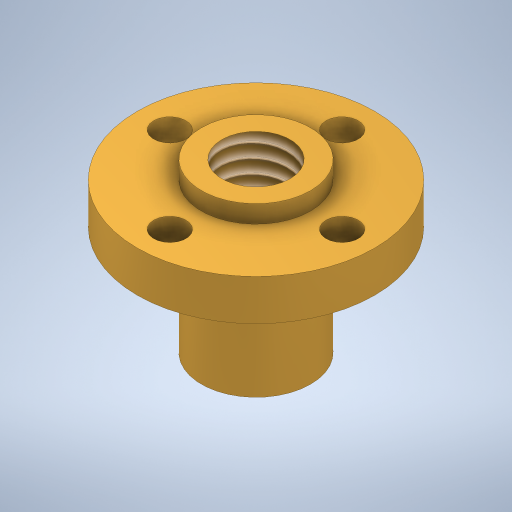
# Autodesk Inventor part: Threaded Rod Mount
Saved by Autodesk Inventor 2024 (Build 280153000, 153)
## iProperties
Created: 2023-06-07
Part Number: Threaded Rod Mount
Material: Generic
Document SubType Name: Modeling
Designer: 18179
Density: 1 g/cm^3
Appearance: Brass - Satin
Author: 18179
Autodesk Inventor part; units mm, degrees
ref_plane "YZ Plane" through (0, 0, 0) normal (1, 0, 0) x (0, 1, 0)
ref_plane "XZ Plane" through (0, 0, 0) normal (0, 1, 0) x (-1, 0, 0)
ref_plane "XY Plane" through (0, 0, 0) normal (0, 0, 1) x (1, 0, 0)
sketch "Sketch1" plane through (0, 0, 0) normal (0, 1, 0) x (-1, 0, 0)
  circle A0 centre (0, 0) radius 11.049
  circle A1 centre (0, 0) radius 3.175
  circle A2 centre (8.025, 0) radius 1.5
  line L0 (9.525, 0) -> (11.049, 0)
  circle A3 centre (0, 0) radius 5.08
  circle A4 centre (0, 8.025) radius 1.5
  circle A5 centre (-8.025, 0) radius 1.5
  circle A6 centre (0, -8.025) radius 1.5
  point P0 (0, 9.525)
  point P1 (-9.525, 0)
  point P2 (0, -9.525)
  dimension "d0" = 22.098
  dimension "d2" = 3
  dimension "d1" = 6.35
  dimension "d3" = 1.524
  dimension "d4" = 10.16
  dimension "d7" = 360
  constraints: 3 coincident, 3 horizontal alignment, 2 centre point, 2 end point, 2 vertical alignment, 1 horizontal, 23 other
  measures "d1" diameter of A1
  measures "d3" distance of L0.start L0.end
  measures "d4" diameter of A3
extrude "Extrusion1" add sketch "Sketch1" along normal blind 3.81 contours A0 | A3
sketch "Sketch2" plane through (0, 3.81, 0) normal (0, 1, 0) x (1, 0, 0)
  circle A0 centre (0, 0) radius 5.08
  circle A1 centre (0, 0) radius 3.175
  dimension "d11" = 10.16
  constraints: 2 centre point, 2 coincident
  measures "d11" diameter of A0
extrude "Extrusion2" add sketch "Sketch2" along normal blind 1.651
sketch "Sketch3" plane through (0, 0, 0) normal (0, -1, 0) x (1, 0, 0)
  circle A0 centre (0, 0) radius 5.08 projected
  circle A1 centre (0, 0) radius 5.08 projected
  circle A2 centre (0, 0) radius 3.175 projected
extrude "Extrusion3" add sketch "Sketch3" along normal blind 10.16
thread "Thread1" size "1/4-20 UNC" class "2B" standard "ANSI Unified Screw Threads" full length
body "Solid1"
